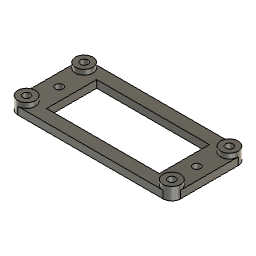
Zero4U Hub Mount v1 (Autodesk Fusion 360 design; units mm, degrees)
Autodesk Fusion 360 part; units mm, degrees
sketch "Sketch1" plane through (0, 0, 0) normal (0, 0, 1) x (1, 0, 0)
  line L0 (-32.5, 15) -> (32.5, 15)
  line L1 (32.5, 15) -> (32.5, -15)
  line L2 (32.5, -15) -> (-32.5, -15)
  line L3 (-32.5, -15) -> (-32.5, 15)
  line L4 (-32.5, 15) -> (32.5, -15) construction
  line L5 (32.5, 15) -> (-32.5, -15) construction
  circle A0 centre (-29, 11.5) radius 1.5
  circle A1 centre (29, 11.5) radius 1.5
  circle A2 centre (-29, -11.5) radius 1.5
  circle A3 centre (29, -11.5) radius 1.5
  dimension "d1" = 65
  dimension "d2" = 30
  dimension "d3" = 3
  dimension "d4" = 3.5
  dimension "d5" = 3.5
  dimension "d8" = 58
  dimension "d9" = -23
  constraint horizontal L0
  constraint perpendicular L0 L1
  constraint parallel L0 L2
  constraint parallel L1 L3
  constraint coincident L4 origin
  constraint coincident L5 origin
  measures "d1" distance of L1.end L2.end
  measures "d2" distance of L0.end L1.end
  measures "d3" diameter of A0
  measures "d4" distance of L0 A0.centre
  measures "d5" distance of L3 A0.centre
extrude "Extrude1" add sketch "Sketch1" along normal blind 3
sketch "Sketch2" plane through (0, 0, 3) normal (0, 0, 1) x (-1, 0, 0)
  circle A0 centre (-29, -11.5) radius 1.5
  circle A1 centre (29, 11.5) radius 1.5
  circle A2 centre (29, -11.5) radius 1.5
  circle A3 centre (-29, 11.5) radius 1.5
  line L0 (32.5, 15) -> (-32.5, 15)
  line L1 (-32.5, 15) -> (-32.5, -15)
  line L2 (-32.5, -15) -> (32.5, -15)
  line L3 (32.5, -15) -> (32.5, 15)
  circle A4 centre (29, -11.5) radius 3.5
  circle A5 centre (-29, -11.5) radius 3.5
  circle A6 centre (29, 11.5) radius 3.5
  circle A7 centre (-29, 11.5) radius 3.5
  dimension "d14" = -58
  dimension "d15" = 23
  constraint concentric A2 A4
  constraint tangent L2 A4
extrude "Extrude2" add sketch "Sketch2" along normal blind 2 contours A6 | A7 | A4 | A5
fillet "Fillet1" radius 3.5 4 edges at (-32.5, -15, 1.5) (-32.5, 15, 1.5) (32.5, -15, 1.5) (32.5, 15, 1.5)
sketch "Sketch3" plane through (0, 0, 3) normal (0, 0, 1) x (-1, 0, 0)
  arc A0 (-29, -15) -> (-32.5, -11.5) centre (-29, -11.5) ccw
  line L0 (-29, -15) -> (29, -15)
  arc A1 (32.5, -11.5) -> (29, -15) centre (29, -11.5) ccw
  line L1 (32.5, -11.5) -> (32.5, 11.5)
  arc A2 (29, 15) -> (32.5, 11.5) centre (29, 11.5) ccw
  line L2 (29, 15) -> (-29, 15)
  arc A3 (-32.5, 11.5) -> (-29, 15) centre (-29, 11.5) ccw
  line L3 (-32.5, 11.5) -> (-32.5, -11.5)
  line L4 (25.5013, -11.5936) -> (-25.5013, 11.5936) construction
  line L5 (-25.5013, -11.5936) -> (25.5013, 11.5936) construction
  circle A4 centre (27.5, 0) radius 1.5
  circle A5 centre (-27.5, 0) radius 1.5
  line L6 (22.5, -10) -> (-22.5, -10)
  line L7 (-22.5, -10) -> (-22.5, 10)
  line L8 (-22.5, 10) -> (22.5, 10)
  line L9 (22.5, 10) -> (22.5, -10)
  line L10 (22.5, -10) -> (-22.5, 10) construction
  line L11 (-22.5, -10) -> (22.5, 10) construction
  dimension "d20" = 3
  dimension "d21" = 3
  dimension "d22" = 27.5
  dimension "d23" = 27.5
  dimension "d24" = 5
  dimension "d25" = 5
  dimension "d26" = 5
  constraint coincident L4 origin
  constraint coincident L5 origin
  constraint coincident A1 L4.start
  constraint horizontal L6
  constraint perpendicular L6 L7
  constraint parallel L6 L8
  constraint parallel L7 L9
  constraint coincident L10 origin
  constraint coincident L11 origin
  measures "d20" diameter of A4
  measures "d21" diameter of A5
  measures "d22" distance of origin A5.centre
  measures "d23" distance of origin A4.centre
  measures "d24" distance of A4.centre L9
  measures "d25" distance of L1 A4.centre
  measures "d26" distance of L2 L8
extrude "Extrude3" cut sketch "Sketch3" against normal up to surface (3 mm away) contours A4 | A5 | L6 L7 L8 L9
equation "d24 = d25"
equation "d26 = d25"
